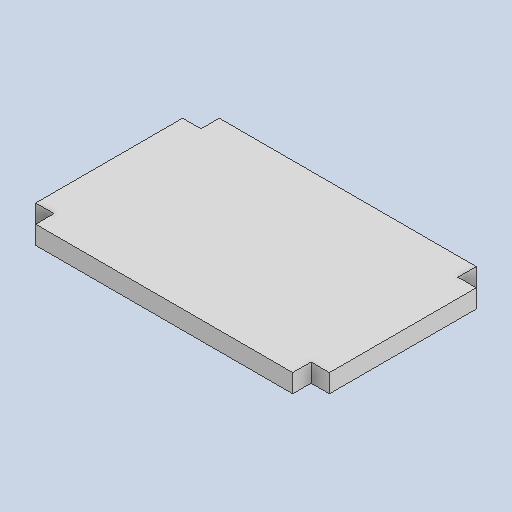
# Autodesk Inventor part: Moving Carousel Wall
Saved by Autodesk Inventor 2023 (Build 270158000, 158)
## iProperties
Created: 2023-02-14
Part Number: Moving Carousel Wall
Material: Generic
Document SubType Name: Modeling
Designer: cheng
Density: 1 g/cm^3
Appearance: Default
Author: cheng
Autodesk Inventor part; units mm, degrees
ref_plane "YZ Plane" through (0, 0, 0) normal (1, 0, 0) x (0, 1, 0)
ref_plane "XZ Plane" through (0, 0, 0) normal (0, 1, 0) x (-1, 0, 0)
ref_plane "XY Plane" through (0, 0, 0) normal (0, 0, 1) x (1, 0, 0)
sketch "Sketch1" plane through (0, 0, 0) normal (0, 1, 0) x (-1, 0, 0)
  line L0 (35, 25) -> (-35, 25)
  line L1 (-35, 25) -> (-35, -25)
  line L2 (-35, -25) -> (35, -25)
  line L3 (35, -25) -> (35, 25)
  line L4 (35, 25) -> (-35, -25) construction
  line L5 (-35, 25) -> (35, -25) construction
  line L6 (40, -20) -> (35, -20)
  line L7 (35, -20) -> (35, 20)
  line L8 (35, 20) -> (40, 20)
  line L9 (40, 20) -> (40, -20)
  line L10 (40, -20) -> (35, 20) construction
  line L11 (35, -20) -> (40, 20) construction
  line L12 (-35, -20) -> (-40, -20)
  line L13 (-40, -20) -> (-40, 20)
  line L14 (-40, 20) -> (-35, 20)
  line L15 (-35, 20) -> (-35, -20)
  line L16 (-35, -20) -> (-40, 20) construction
  line L17 (-40, -20) -> (-35, 20) construction
  line L18 (35, 0) -> (0, 0)
  line L19 (37.5, 0) -> (40, 0) construction
  line L20 (-37.5, 0) -> (-35, 0) construction
  point P0 (35, -20)
  point P1 (-35, 20)
  point P2 (-35, -20)
  dimension "d0" = 5
  dimension "d1" = 5
  dimension "d2" = 40
  dimension "d3" = 50
  dimension "d4" = 40
  dimension "d5" = 70
  constraints: 42 end point, 8 midpoint, 6 parallel, 4 collinear, 4 perpendicular, 3 horizontal
  measures "d0" distance of L12.start L12.end
  measures "d1" distance between parallel lines of L7 L9
  measures "d2" distance between parallel lines of L6 L8
  measures "d3" distance between parallel lines of L2 L0
  measures "d4" distance between parallel lines of L12 L14
  measures "d5" distance between parallel lines of L15 L3
extrude "Extrusion1" add sketch "Sketch1" along normal blind 5
body "Solid1"
